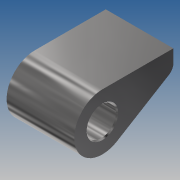
# Autodesk Inventor part: DD_KVD_003_10_A
Saved by Autodesk Inventor 2017.3 (Build 213256000, 256)
## iProperties
Created: 2023-12-12
Part Number: DD_KVD_003_10_A
Material: Nerezová ocel
Document SubType Name: Modeling
Designer: Darena
Manufacturer: Standard
Standards Organization: Custom
Density: 8 g/cm^3
Appearance: Pololeštěná
Author: Darena
Autodesk Inventor part; units mm, degrees
ref_plane "YZ Plane" through (0, 0, 0) normal (1, 0, 0) x (0, 1, 0)
ref_plane "XZ Plane" through (0, 0, 0) normal (0, 1, 0) x (-1, 0, 0)
ref_plane "XY Plane" through (0, 0, 0) normal (0, 0, 1) x (1, 0, 0)
sketch "Náčrt2" plane through (0, 0, 0) normal (1, 0, 0) x (0, 1, 0)
  circle A0 centre (0, 0) radius 6.5
  line L0 (31.5, 12.5) -> (0, 12.5)
  line L1 (31.5, 12.5) -> (31.5, 4.5)
  line L2 (31.5, 4.5) -> (6.4868, -10.6851)
  arc A1 (0, 12.5) -> (6.4868, -10.6851) centre (0, 0) ccw
  dimension "d0" = 13
  dimension "d1" = 6
  dimension "d2" = 31.5
  dimension "d3" = 8
  constraints: 6 end point, 2 centre point, 2 coincident, 2 point on circle, 2 tangent, 1 horizontal, 1 vertical
  measures "d0" diameter of A0
  measures "d1" radial gap between concentric circles of A0 A1
  measures "d2" distance of L0.start L0.end
  measures "d3" distance of L0.start L1.end
extrude "Vysunutí1" add sketch "Náčrt2" along normal blind 30
fillet "Zaoblení1" radius 4 1 edges at (15, 31.5, 4.5)
chamfer "Zkosení1" distance 0.5 angle 45 2 edges at (0, -6.5, 0) (30, -6.5, 0)
